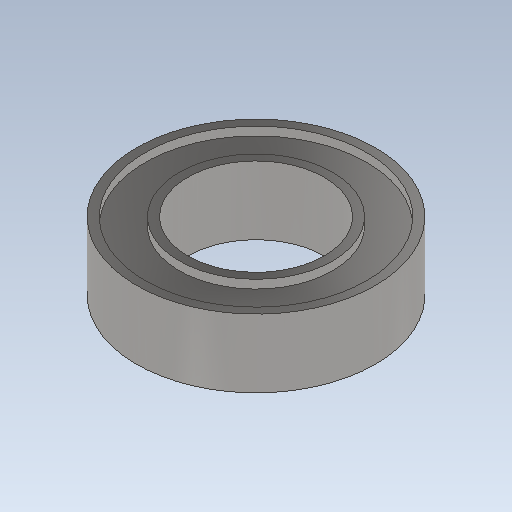
# Autodesk Inventor part: Подшипник 8х14х4
Saved by Autodesk Inventor 2021.1 (Build 251245010, 245A)
## iProperties
Created: 2025-12-07
Part Number: Подшипник 8х14х4
Material: Типовые
Document SubType Name: Modeling
Designer: Андрей Тарасов
Density: 1 g/cm^3
Appearance: По умолчанию
Author: Андрей Тарасов
Autodesk Inventor part; units mm, degrees
ref_plane "YZ Plane" through (0, 0, 0) normal (1, 0, 0) x (0, 1, 0)
ref_plane "XZ Plane" through (0, 0, 0) normal (0, 1, 0) x (-1, 0, 0)
ref_plane "XY Plane" through (0, 0, 0) normal (0, 0, 1) x (1, 0, 0)
sketch "Эскиз1" plane through (0, 0, 0) normal (0, 0, 1) x (1, 0, 0)
  line L0 (7, -2) -> (-7, -2)
  line L1 (-7, -2) -> (-7, 2)
  line L2 (-7, 2) -> (7, 2)
  line L3 (7, 2) -> (7, -2)
  line L4 (7, -2) -> (-7, 2) construction
  line L5 (-7, -2) -> (7, 2) construction
  line L6 (4, -2) -> (-4, -2)
  line L7 (-4, -2) -> (-4, 2)
  line L8 (-4, 2) -> (4, 2)
  line L9 (4, 2) -> (4, -2)
  line L10 (4, -2) -> (-4, 2) construction
  line L11 (-4, -2) -> (4, 2) construction
  line L12 (6.5, -1.5) -> (4.5, -1.5)
  line L13 (4.5, -2) -> (4.5, 2)
  line L14 (4.5, 1.5) -> (6.5, 1.5)
  line L15 (6.5, 2) -> (6.5, -2)
  line L16 (6.5, -1.5) -> (4.5, 1.5) construction
  line L17 (4.5, -1.5) -> (6.5, 1.5) construction
  line L18 (0, -2) -> (0, 2) construction
  point P0 (0, 0)
  point P1 (5.5, 0)
  dimension "d1" = 14
  dimension "d2" = 8
  dimension "d3" = 4
  dimension "d4" = 0.5
  dimension "d5" = 0.5
  dimension "d6" = 0.5
  dimension "d7" = 0.5
  constraints: 38 end point, 8 midpoint, 8 point on line, 6 parallel, 3 horizontal, 3 perpendicular, 1 collinear
  measures "d1" distance between parallel lines of L3 L1
  measures "d2" distance between parallel lines of L9 L7
  measures "d3" distance between parallel lines of L0 L2
  measures "d4" distance between parallel lines of L3 L15
  measures "d5" distance between parallel lines of L13 L9
  measures "d6" distance between parallel lines of L2 L14
  measures "d7" distance between parallel lines of L0 L12
revolve "Вращение1" add sketch "Эскиз1" angle 360 about axis through (0, -2, 0) along (0, 1, 0) contours L0 L15 L2 L3 | L0 L9 L2 L13 | L12 L13 L14 L15
equation "\"d4\" = d6"
equation "\"d6\" = d7"
equation "\"d7\" = d5"
